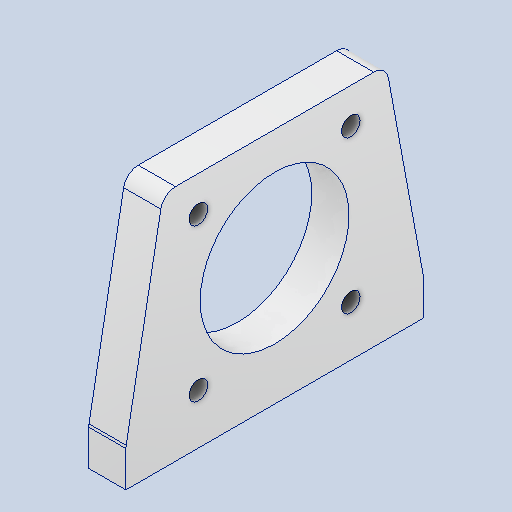
# Autodesk Inventor part: belt_liner_v5_Plate_12
Saved by Autodesk Inventor 2025.2 (Build 292293000, 293)
## iProperties
Created: 2025-02-23
Part Number: belt_liner_v5_Plate_12
Material: アルミニウム 6061
Document SubType Name: Modeling
Designer: haruy
Density: 2.7 g/cm^3
Appearance: アルミニウム - フラット
Author: haruy
Autodesk Inventor part; units mm, degrees
ref_plane "YZ Plane" through (0, 0, 0) normal (1, 0, 0) x (0, 1, 0)
ref_plane "XZ Plane" through (0, 0, 0) normal (0, 1, 0) x (-1, 0, 0)
ref_plane "XY Plane" through (0, 0, 0) normal (0, 0, 1) x (1, 0, 0)
sketch "スケッチ1" plane through (0, 0, 0) normal (1, 0, 0) x (0, 1, 0)
  line L0 (0, 0) -> (30, 0)
  line L1 (30, 0) -> (30, -30)
  line L2 (30, -30) -> (0, -30)
  line L3 (0, -30) -> (0, 0)
  circle A0 centre (25.253, -4.747) radius 1.25
  line L4 (15, 0) -> (15, -30)
  line L5 (30, -15) -> (0, -15)
  circle A1 centre (4.747, -4.747) radius 1.25
  circle A2 centre (25.253, -25.253) radius 1.25
  circle A3 centre (4.747, -25.253) radius 1.25
  line L6 (-2, 5) -> (3, 5)
  line L7 (3, 5) -> (3, -35)
  line L8 (3, -35) -> (-2, -35)
  line L9 (-2, -35) -> (-2, 5)
  line L10 (30, 0) -> (3, 5)
  line L11 (30, -30) -> (3, -35)
  circle A4 centre (15, -15) radius 10
  dimension "d0" = 30
  dimension "d1" = 30
  dimension "d2" = 2.5
  dimension "d3" = 4.747
  dimension "d4" = 4.747
  dimension "d5" = 5
  dimension "d6" = 2
  dimension "d7" = 5
  dimension "d8" = 5
  dimension "d12" = 20
  constraints: 24 end point, 5 centre point, 5 midpoint, 4 parallel, 3 symmetric about line, 2 horizontal, 2 perpendicular, 3 other
  measures "d0" distance of L1.end L2.end
  measures "d1" distance of L0.end L1.end
  measures "d2" diameter of A0
  measures "d3" distance from line of A0.centre L1
  measures "d4" distance from line of L0 A0.centre
  measures "d5" distance of L7.end L8.end
  measures "d6" distance between parallel lines of L3 L9
  measures "d7" distance between parallel lines of L6 L0
  measures "d8" distance between parallel lines of L8 L2
  measures "d12" diameter of A4
extrude "押し出し1" add sketch "スケッチ1" against normal blind 5 contours L0 L7 L10 | L4 A4 L5 L7 L0 | L0 L1 L5 A4 L4 | L7 L5 L3 L0 | L0 L3 L2 L7 L8 L9 L6 | L1 L2 L4 A4 L5 | L7 L2 L3 L5 | L5 A4 L4 L2 L7 | L11 L7 L2
fillet "フィレット1" radius 2 4 edges at (-2.5, 30, 0) (-2.5, 3, 5) (-2.5, 30, -30) (-2.5, 3, -35)
sketch "スケッチ2" plane through (0, -2, -35) normal (0, -1, 0) x (1, 0, 0)
  line L0 (0, 0) -> (-5, 0) projected
  line L1 (-2.5, 0) -> (-2.5, 40)
  line L2 (0, 40) -> (-5, 40) projected
  point P0 (0, 35)
  point P1 (-2.5, 15)
  point P2 (-2.5, 25)
  dimension "d13" = 15
  dimension "d14" = 10
  constraints: 2 end point, 2 midpoint, 2 point on line
  measures "d13" distance from line of L0 point (-2.5, 15)
  measures "d14" distance of point (-2.5, 15) point (-2.5, 25)
hole "穴1" at (-2.5, -2, -20) at (-2.5, -2, -10) direction (0, 1, 0) diameter 2.5 depth 5 tip angle 118
equation "\"d4\" = d3"
